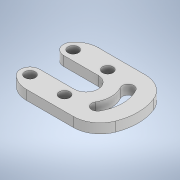
# Autodesk Inventor part: Part7
Saved by Autodesk Inventor 2021 (Build 250183000, 183)
## iProperties
Created: 2022-04-24
Part Number: Part7
Material: Generic
Document SubType Name: Modeling
Designer: hp
Density: 1 g/cm^3
Appearance: Default
Author: hp
Autodesk Inventor part; units mm, degrees
ref_plane "YZ Plane" through (0, 0, 0) normal (1, 0, 0) x (0, 1, 0)
ref_plane "XZ Plane" through (0, 0, 0) normal (0, 1, 0) x (-1, 0, 0)
ref_plane "XY Plane" through (0, 0, 0) normal (0, 0, 1) x (1, 0, 0)
sketch "Sketch1" plane through (0, 0, 0) normal (0, 1, 0) x (-1, 0, 0)
  arc A0 (-50.2663, 19.7308) -> (-50.2663, -19.7308) centre (0, 0) ccw
  line L0 (24.8197, 37.5) -> (-24.2023, 37.5)
  line L1 (-24.2023, -37.5) -> (24.8197, -37.5)
  circle A1 centre (0, 0) radius 12.5
  circle A2 centre (0, -22.5) radius 5.5
  circle A3 centre (0, 22.5) radius 5.5
  arc A4 (-24.2023, 37.5) -> (-50.2663, 19.7308) centre (-24.2023, 9.5) ccw
  line L2 (-14, 0) -> (-38, 0)
  arc A5 (-50.2663, -19.7308) -> (-24.2023, -37.5) centre (-24.2023, -9.5) ccw
  line L3 (0, 0) -> (-36.2595, -20.9344)
  line L4 (0, 0) -> (-38.6065, 22.2895)
  circle A6 centre (-27.7128, 16) radius 6
  circle A7 centre (-27.7128, -16) radius 6
  arc A8 (-22.5167, 13) -> (-22.5167, -13) centre (0, 0) ccw
  arc A9 (-32.909, 19) -> (-32.909, -19) centre (0, 0) ccw
  line L5 (38.0847, -33.6906) -> (38.0847, -32.2803)
  line L6 (38.0847, 32.2803) -> (38.0847, 33.6906)
  arc A10 (36, 12.5) -> (43.4536, 29.1667) centre (36, 22.5) ccw
  arc A11 (43.4536, -29.1667) -> (36, -12.5) centre (36, -22.5) ccw
  line L7 (0, 12.5) -> (0, -12.5)
  arc A12 (3.9746, 26.3016) -> (3.6179, 25.7471) centre (24.8197, 12.5) ccw
  arc A13 (-0.1803, 12.4987) -> (0, 9.5026) centre (24.8197, 12.5) ccw
  arc A14 (1.3171, -21.0223) -> (3.9746, -26.3016) centre (24.8197, -12.5) ccw
  arc A15 (24.8197, -37.5) -> (43.4536, -29.1667) centre (24.8197, -12.5) ccw
  arc A16 (0, -9.5026) -> (-0.1803, -12.4987) centre (24.8197, -12.5) ccw
  arc A17 (43.4536, 29.1667) -> (24.8197, 37.5) centre (24.8197, 12.5) ccw
  line L8 (0, 12.5) -> (36, 12.5)
  line L9 (49.8197, 12.5) -> (55, 12.5)
  line L10 (0, -12.5) -> (36, -12.5)
  line L11 (49.8197, -12.5) -> (57, -12.5)
  arc A18 (24.8197, -12.5) -> (29.6533, -12.0283) centre (24.8197, 12.5) ccw
  arc A19 (36.8095, -9.4373) -> (38.0847, -8.6906) centre (24.8197, 12.5) ccw
  arc A20 (-24.2389, 20.892) -> (-27.7128, 16) centre (0, 0) ccw
  arc A21 (-30.2125, -10.5455) -> (-24.2389, -20.892) centre (0, 0) ccw
  circle A22 centre (36, 22.5) radius 5.5
  circle A23 centre (36, -22.5) radius 5.5
  dimension "d5" = 11
  dimension "d6" = 11
  dimension "d0" = 108
  dimension "d4" = 25
  dimension "d7" = 45
  dimension "d8" = 22.5
  dimension "d9" = 37.5
  dimension "d10" = 37.5
  dimension "d13" = 30
  dimension "d14" = 30
  dimension "d15" = 12
  dimension "d16" = 12
  dimension "d17" = 20
  dimension "d18" = 20
  dimension "d19" = 36
  dimension "d20" = 36
  dimension "d23" = 11
  dimension "d24" = 11
  constraints: 51 point on circle, 24 end point, 22 centre point, 9 coincident, 7 point on line, 6 tangent, 5 horizontal, 3 symmetric about line, 1 parallel, 1 vertical, 7 other
  measures "d0" diameter of A0
  measures "d4" diameter of A1
  measures "d7" distance of point (0, 22.5) point (0, -22.5)
  measures "d8" distance of point (0, 22.5) point (0, 0)
  measures "d9" distance from line of L1 point (0, 0)
  measures "d10" distance from line of point (0, 0) L0
  measures "d13" angle of L2 L3
  measures "d14" angle of L4 L2
  measures "d15" diameter of A6
  measures "d16" diameter of A7
  measures "d17" diameter of A10
  measures "d18" diameter of A11
  measures "d19" distance of point (0, 22.5) A10.centre
  measures "d20" distance of point (0, -22.5) A11.centre
  measures "d23" diameter of A22
  measures "d24" diameter of A23
extrude "Extrusion1" add sketch "Sketch1" along normal blind 10 contours A4 L0 A17 A10 L8 A1 L4 A6 A9 A7 L3 L10 A11 A15 L1 A5 A0 | A1 L3 A8 L4
equation "\"d5\" = d6"
equation "\"d8\" = 0.5 * d7"
equation "\"d9\" = 0.5 * d1"
equation "\"d10\" = d9"
equation "\"d16\" = d15"
equation "\"d18\" = d17"
equation "\"d1\" = 75"
body "Solid1"
